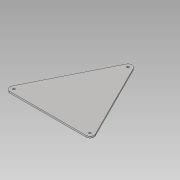
# Autodesk Inventor part: Bed Support
Saved by Autodesk Inventor 2016 (Build 200138000, 138)
## iProperties
Created: 2017-05-19
Part Number: Bed Support
Material: Generic
Document SubType Name: Modeling
Designer: 31745
Density: 1 g/cm^3
Appearance: Default
Author: 31745
Autodesk Inventor part; units mm, degrees
ref_plane "YZ Plane" through (0, 0, 0) normal (1, 0, 0) x (0, 1, 0)
ref_plane "XZ Plane" through (0, 0, 0) normal (0, 1, 0) x (-1, 0, 0)
ref_plane "XY Plane" through (0, 0, 0) normal (0, 0, 1) x (1, 0, 0)
sketch "Sketch1" plane through (0, 0, 0) normal (0, 1, 0) x (-1, 0, 0)
  line L0 (76.2, 0) -> (-76.2, 0)
  line L1 (0, 0) -> (0, -152.4)
  line L2 (7.0995, -155.9498) -> (83.2995, -3.5498)
  line L3 (76.2, 7.9375) -> (-76.2, 7.9375)
  line L4 (-83.2995, -3.5498) -> (-7.0995, -155.9498)
  circle A0 centre (76.2, 0) radius 7.9375
  circle A1 centre (-76.2, 0) radius 7.9375
  circle A2 centre (0, -152.4) radius 7.9375
  dimension "d0" = 152.4
  dimension "d1" = 152.4
  dimension "d3" = 15.875
  dimension "d4" = 15.875
  dimension "d5" = 15.875
  constraints: 10 end point, 6 point on circle, 5 tangent, 4 coincident, 3 centre point, 3 horizontal, 1 midpoint, 1 vertical
  measures "d0" distance of L1.start L1.end
  measures "d1" distance of L0.end L0.start
  measures "d3" diameter of A0
  measures "d4" diameter of A1
  measures "d5" diameter of A2
extrude "Extrusion1" add sketch "Sketch1" along normal blind 3.175
sketch "Sketch2" plane through (0, 3.175, 0) normal (0, 1, 0) x (1, 0, 0)
  arc A0 (-83.2995, 3.5498) -> (-76.2, -7.9375) centre (-76.2, 0) ccw projected
  line L0 (-76.2, -7.9375) -> (76.2, -7.9375) projected
  arc A1 (76.2, -7.9375) -> (83.2995, 3.5498) centre (76.2, 0) ccw projected
  line L1 (83.2995, 3.5498) -> (7.0995, 155.9498) projected
  arc A2 (7.0995, 155.9498) -> (-7.0995, 155.9498) centre (0, 152.4) ccw projected
  line L2 (-7.0995, 155.9498) -> (-83.2995, 3.5498) projected
  point P0 (0, 0)
hole "Hole1" at (-76.2, 3.175, 0) at (76.2, 3.175, 0) at (0, 3.175, -152.4) direction (0, -1, 0) diameter 4.4958 end through all clearance for "Countersunk Flat Head Screw ISO 2009/7046" size "M4" standard "ISO"
body "Solid1"
